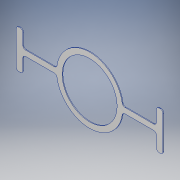
# Autodesk Inventor part: Frame
Saved by Autodesk Inventor 2019 (Build 230136000, 136)
## iProperties
Created: 2020-03-05
Part Number: Frame
Material: Aluminum 6061
Document SubType Name: Sheet Metal
Designer: student
Density: 2.7 g/cm^3
Sheet Metal Rule: Default
Appearance: Aluminum - Flat
Flat Pattern Width: 16.9342 cm
Flat Pattern Length: 7.62 cm
Flat Pattern Area: 129.038 cm^2
Sheet Metal Width: 6.667 in
Sheet Metal Length: 3.000 in
Sheet Metal Area: 20.001 in^2
Author: student
Autodesk Inventor part; units mm, degrees
ref_plane "YZ Plane" through (0, 0, 0) normal (1, 0, 0) x (0, 1, 0)
ref_plane "XZ Plane" through (0, 0, 0) normal (0, 1, 0) x (-1, 0, 0)
ref_plane "XY Plane" through (0, 0, 0) normal (0, 0, 1) x (1, 0, 0)
sketch "Sketch1" plane through (0, 0, 0) normal (0, 0, 1) x (1, 0, 0)
  circle A0 centre (0, 0) radius 38.1
  circle A1 centre (0, 0) radius 31.75
  line L0 (-84.6709, -3.175) -> (-84.6709, 3.175)
  line L1 (84.6709, 3.175) -> (84.6709, -3.175)
  line L2 (84.6709, -3.175) -> (-84.6709, 3.175) construction
  line L3 (-84.6709, -3.175) -> (84.6709, 3.175) construction
  line L4 (84.6709, -3.175) -> (37.9675, -3.175)
  line L5 (-37.9675, -3.175) -> (-84.6709, -3.175)
  line L6 (-84.6709, 3.175) -> (-37.9675, 3.175)
  line L7 (37.9675, 3.175) -> (84.6709, 3.175)
  line L8 (-84.6709, 22.225) -> (-77.0509, 22.225)
  line L9 (-77.0509, 22.225) -> (-77.0509, -22.225)
  line L10 (-77.0509, -22.225) -> (-84.6709, -22.225)
  line L11 (-84.6709, -22.225) -> (-84.6709, 22.225)
  line L12 (0, 31.75) -> (0, -31.75) construction
  line L13 (84.6709, 22.225) -> (77.0509, 22.225)
  line L14 (77.0509, 22.225) -> (77.0509, -22.225)
  line L15 (77.0509, -22.225) -> (84.6709, -22.225)
  line L16 (84.6709, -22.225) -> (84.6709, 22.225)
  dimension "d0" = 76.2
  dimension "d1" = 6.35
  dimension "d2" = 169.3418
  dimension "d4" = 6.35
  dimension "d5" = 19.05
  dimension "d6" = 19.05
  dimension "d7" = 7.62
  measures "d0" diameter of A0
  measures "d1" radial gap between concentric circles of A0 A1
  measures "d2" distance of L0.end L1.start
  measures "d4" distance between parallel lines of L5 L6
  measures "d5" distance between parallel lines of L10 L5
  measures "d6" distance between parallel lines of L6 L8
  measures "d7" distance of L8.start L8.end
extrude "Plate1" add sketch "Sketch1" along normal blind 0.889
fillet "Corner Round1" radius 3.175 16 edges at (77.0509, -3.175, 0.4445) (77.0509, -22.225, 0.4445) (77.0509, 3.175, 0.4445) (77.0509, 22.225, 0.4445) (84.6709, -22.225, 0.4445) (84.6709, 22.225, 0.4445) (37.9675, -3.175, 0.4445) (-77.0509, -3.175, 0.4445) (-77.0509, -22.225, 0.4445) (-77.0509, 3.175, 0.4445) (-77.0509, 22.225, 0.4445) (-84.6709, -22.225, 0.4445) (-84.6709, 22.225, 0.4445) (-37.9675, 3.175, 0.4445) (-37.9675, -3.175, 0.4445) (37.9675, 3.175, 0.4445)
equation "\"d8\" = Thickness"
equation "\"BendRadius\" = Thickness"
equation "\"BendReliefWidth\" = Thickness"
equation "\"BendReliefDepth\" = 0.5 * Thickness"
equation "\"CornerReliefSize\" = 4 * Thickness"
equation "\"MinimumRemnant\" = 2 * Thickness"
equation "\"TransitionRadius\" = BendRadius"
equation "\"JacobiRadiusSize\" = Thickness"
equation "\"GapSize\" = Thickness"
equation "\"Thickness\" = 0.889"
body "Solid1"
